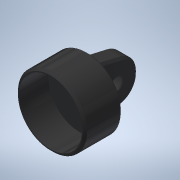
# Autodesk Inventor part: shocks_fixed
Saved by Autodesk Inventor 2020 (Build 240168000, 168)
## iProperties
Created: 2015-12-04
Part Number: shocks_fixed
Material: Goma
Document SubType Name: Modeling
Designer: MIGUEL ANGEL
Density: 0.93 g/cm^3
Appearance: Goma - Negro - Versión 1.1
Author: MIGUEL ANGEL
Autodesk Inventor part; units mm, degrees
ref_plane "YZ Plane" through (0, 0, 0) normal (1, 0, 0) x (0, 1, 0)
ref_plane "XZ Plane" through (0, 0, 0) normal (0, 1, 0) x (-1, 0, 0)
ref_plane "XY Plane" through (0, 0, 0) normal (0, 0, 1) x (1, 0, 0)
sketch "Boceto1" plane through (0, 0, 0) normal (0, 1, 0) x (-1, 0, 0)
  circle A0 centre (0, 0) radius 16.5
  dimension "d0" = 33
  constraints: 1 centre point, 1 coincident
  measures "d0" diameter of A0
extrude "Extrusión1" add sketch "Boceto1" along normal blind 18
sketch "Boceto3" plane through (0, 0, 0) normal (1, 0, 0) x (0, 1, 0)
  line L0 (18, -16.5) -> (18, 16.5) projected
  line L1 (18, -12.5) -> (30, -9.7467)
  arc A0 (30, -9.7467) -> (37.7637, 0) centre (27.7637, 0) ccw
  line L2 (18, 0) -> (51.6641, 0)
  line L3 (18, 12.5) -> (30, 9.7467)
  arc A1 (37.7637, 0) -> (30, 9.7467) centre (27.7637, 0) ccw
  line L4 (18, 12.5) -> (18, -12.5)
  point P0 (0, 0)
  dimension "d5" = 10
  dimension "d6" = 4
  dimension "d7" = 12
  constraints: 8 end point, 4 point on circle, 2 centre point, 2 point on line, 2 symmetric about line, 1 collinear, 1 horizontal, 1 horizontal alignment, 1 midpoint, 1 tangent, 1 other
  measures "d5" radius of A0
  measures "d6" distance of L0.start L1.start
  measures "d7" horizontal distance of L1.start L1.end
extrude "Extrusión2" add sketch "Boceto3" along normal mid plane 8
sketch "Boceto4" plane through (4, 0, 0) normal (1, 0, 0) x (0, 0, -1)
  arc A0 (9.7467, 30) -> (-9.7467, 30) centre (0, 27.7637) ccw projected
  circle A1 centre (0, 27.7637) radius 3
  point P0 (0, 0)
  dimension "d10" = 6
  constraints: 1 centre point, 1 coincident
  measures "d10" diameter of A1
extrude "Extrusión3" cut sketch "Boceto4" against normal through all
sketch "Boceto6" plane through (0, 0, 0) normal (0, -1, 0) x (1, 0, 0)
  circle A0 centre (0, 0) radius 15
  dimension "d14" = 30
  constraints: 1 centre point, 1 coincident
  measures "d14" diameter of A0
extrude "Extrusión4" cut sketch "Boceto6" against normal blind 14
chamfer "Chaflán1" distance 1 angle 45 10 edges at (16.5, 18, 0) (16.5, 0, 0) (-4, 37.7637, 0) (-4, 24, -11.1234) (-4, 24, 11.1234) (4, 37.7637, 0) (4, 24, 11.1234) (4, 24, -11.1234) (0, 18, 12.5) (0, 18, -12.5)
sketch "Boceto7" plane through (0, 0, 0) normal (0, 0, 1) x (1, 0, 0)
  arc A0 (5, 27.7637) -> (-5, 27.7637) centre (0, 27.7637) ccw
  line L0 (4, 36.7637) -> (4, 29.7764) projected
  line L1 (-4, 29.7764) -> (-4, 36.7637) projected
  line L2 (-4, 29.7764) -> (-4, 19.9747) projected
  line L3 (4, 19.9747) -> (4, 29.7764) projected
  line L4 (4, 30.7637) -> (-4, 30.7637) projected
  line L5 (4, 24.7637) -> (-4, 24.7637) projected
  line L6 (8.3579, 27.7637) -> (-7.6994, 27.7637)
  point P0 (0, 0)
  dimension "d20" = 5
  constraints: 4 point on circle, 3 end point, 2 point on line, 1 centre point, 1 horizontal
  measures "d20" radius of A0
revolve "Revolución1" cut sketch "Boceto7" angle 360 about axis through (8.3579, 27.7637, 0) along (-1, 0, 0) contours L6 L3 L0 A0 | L4 A0 | L0 L3 L6 L2 L1 L4 | L1 L2 L6 A0
